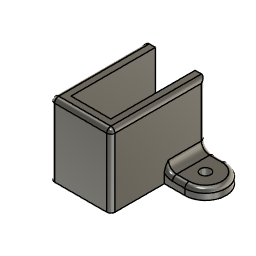
Motor Mount v1 (Autodesk Fusion 360 design; units mm, degrees)
Autodesk Fusion 360 part; units mm, degrees
sketch "Sketch1" plane through (0, 0, 0) normal (0, 0, 1) x (1, 0, 0)
  line L0 (0, 0) -> (12.2682, 0)
  line L1 (12.2682, 0) -> (12.2682, 22.86)
  line L2 (12.2682, 22.86) -> (0, 22.86)
  line L3 (0, 22.86) -> (0, 0)
  line L4 (-3.175, -3.175) -> (15.4432, -3.175)
  line L5 (15.4432, -3.175) -> (15.4432, 26.035)
  line L6 (15.4432, 26.035) -> (-3.175, 26.035)
  line L7 (-3.175, 26.035) -> (-3.175, -3.175)
  line L8 (0, 22.86) -> (0, 26.035)
  line L9 (12.2682, 22.86) -> (12.2682, 26.035)
  dimension "d1" = 12.2682
  dimension "d2" = 22.86
  dimension "d3" = 3.175
  constraint horizontal L0
  constraint vertical L1
  constraint horizontal L2
  constraint vertical L3
  constraint coincident L0.start L3.end
  constraint coincident L6 L8.end
  constraint perpendicular L6 L8
  constraint coincident L6 L9.end
  constraint perpendicular L6 L9
  measures "d1" distance of L0.start L0.end
  measures "d2" distance of L0.start L2.end
extrude "Extrude1" add sketch "Sketch1" along normal blind 3.175
sketch "Sketch2" plane through (0, 0, 3.175) normal (0, 0, 1) x (-1, 0, 0)
  line L0 (3.175, -26.035) -> (3.175, 3.175)
  line L1 (3.175, 3.175) -> (-15.4432, 3.175)
  line L2 (-15.4432, 3.175) -> (-15.4432, -26.035)
  line L3 (-15.4432, -26.035) -> (3.175, -26.035)
  line L4 (-12.2682, 0) -> (-12.2682, -22.86)
  line L5 (-12.2682, -22.86) -> (0, -22.86)
  line L6 (0, -22.86) -> (0, 0)
  line L7 (0, 0) -> (-12.2682, 0)
  dimension "d6" = -3.175
extrude "Extrude2" add sketch "Sketch2" along normal blind 3.175
sketch "Sketch3" plane through (0, 0, 6.35) normal (0, 0, 1) x (-1, 0, 0)
  line L0 (-12.2682, 0) -> (0, 0)
  line L1 (0, 0) -> (0, -22.86)
  line L2 (0, -22.86) -> (-12.2682, -22.86)
  line L3 (-12.2682, -22.86) -> (-12.2682, 0)
  line L4 (-15.4432, -26.035) -> (3.175, -26.035)
  line L5 (3.175, -26.035) -> (3.175, 3.175)
  line L6 (3.175, 3.175) -> (-15.4432, 3.175)
  line L7 (-15.4432, 3.175) -> (-15.4432, -26.035)
  line L8 (0, -22.86) -> (0, -26.035)
  line L9 (-12.2682, -22.86) -> (-12.2682, -26.035)
  constraint coincident L1.end L2.start
  constraint coincident L4 L8.end
  constraint perpendicular L4 L8
  constraint coincident L2.end L3.start
  constraint coincident L4 L9.end
  constraint perpendicular L4 L9
extrude "Extrude3" add sketch "Sketch3" along normal blind 16.002 contours L0 L1 L3 L4 L5 L6 L7 L8 L9
sketch "Sketch4" plane through (0, 0, 0) normal (0, 0, -1) x (1, 0, 0)
  line L0 (-3.175, 3.175) -> (-3.175, -26.035)
  line L1 (-3.175, -26.035) -> (15.4432, -26.035)
  line L2 (15.4432, -26.035) -> (15.4432, 3.175)
  line L3 (15.4432, 3.175) -> (-3.175, 3.175)
  line L4 (15.4432, -26.035) -> (21.7932, -26.035)
  line L5 (21.7932, -26.035) -> (21.7932, -19.685)
  line L6 (21.7932, -19.685) -> (15.4432, -19.685)
  line L7 (15.4432, -19.685) -> (15.4432, -26.035)
  line L8 (-3.175, -26.035) -> (-9.525, -26.035)
  line L9 (-9.525, -26.035) -> (-9.525, -19.685)
  line L10 (-9.525, -19.685) -> (-3.175, -19.685)
  line L11 (-3.175, -19.685) -> (-3.175, -26.035)
  circle A0 centre (21.7932, -19.685) radius 6.35
  circle A1 centre (-9.525, -19.685) radius 6.35
  line L12 (-9.525, -19.685) -> (21.7932, -19.685)
  line L13 (21.7932, -19.685) -> (21.7932, -13.335)
  line L14 (21.7932, -13.335) -> (-9.525, -13.335)
  line L15 (-9.525, -13.335) -> (-9.525, -19.685)
  dimension "d11" = 6.35
  dimension "d12" = 6.35
  dimension "d13" = 6.35
  dimension "d14" = 6.35
  constraint horizontal L4
  constraint vertical L5
  constraint horizontal L6
  constraint vertical L7
  constraint coincident L1.end L2.start
  constraint horizontal L8
  constraint vertical L9
  constraint horizontal L10
  constraint vertical L11
  constraint coincident L0.end L1.start
  constraint coincident L5.end L6.start
  constraint coincident L4.end A0
  constraint coincident L9.end L10.start
  constraint coincident L8.end A1
  constraint horizontal L12
  constraint vertical L13
  constraint horizontal L14
  constraint vertical L15
  constraint coincident A0 L13.end
  measures "d11" distance of L1.end L4.end
  measures "d12" distance of L1.end L6.end
  measures "d13" distance of L0.end L8.end
  measures "d14" distance of L0.end L10.end
extrude "Extrude4" add sketch "Sketch4" against normal blind 3.175 contours L0 A1 L14 | L9 L10 A1 L12 | L10 A1 L12 L15 | L0 L8 L11 A1 | L9 A1 L15 | L2 L4 L7 A0 | L6 A0 L12 L13 | L2 A0 L14 | L5 L6 A0 L12 | L5 A0 L13
sketch "Sketch5" plane through (0, 0, 3.175) normal (0, 0, 1) x (-1, 0, 0)
  line L0 (-15.4432, -26.035) -> (-15.4432, -13.335)
  line L1 (-15.4432, -13.335) -> (-21.7932, -13.335)
  arc A0 (-21.7932, -13.335) -> (-21.7932, -26.035) centre (-21.7932, -19.685) ccw
  line L2 (-21.7932, -26.035) -> (-15.4432, -26.035)
  circle A1 centre (-21.7932, -19.685) radius 1.5875
  dimension "d17" = 3.175
  constraint concentric A0 A1
  measures "d17" diameter of A1
extrude "Extrude5" cut sketch "Sketch5" against normal blind 127 contours A1
sketch "Sketch6" plane through (0, 0, 3.175) normal (0, 0, 1) x (-1, 0, 0)
  arc A0 (9.525, -26.035) -> (9.525, -13.335) centre (9.525, -19.685) ccw
  line L0 (9.525, -13.335) -> (3.175, -13.335)
  line L1 (3.175, -13.335) -> (3.175, -26.035)
  line L2 (3.175, -26.035) -> (9.525, -26.035)
  circle A1 centre (9.525, -19.685) radius 1.5875
  dimension "d20" = 3.175
  constraint concentric A0 A1
  measures "d20" diameter of A1
extrude "Extrude6" cut sketch "Sketch6" against normal blind 25.4 contours A1
fillet "Fillet1" radius 2.54 1 edges at (15.4432, 19.685, 3.175)
fillet "Fillet2" radius 2.54 1 edges at (-3.175, 19.685, 3.175)
fillet "Fillet3" radius 1.27 17 edges at (-3.175, 11.43, 22.352) (-3.9189, 13.335, 3.9189) (-7.62, 13.335, 3.175) (-15.875, 19.685, 3.175) (-7.62, 26.035, 3.175) (-3.9189, 26.035, 3.9189) (-3.175, 26.035, 14.0335) (-3.175, -3.175, 11.176) (15.4432, -3.175, 11.176) (6.1341, -3.175, 22.352) (15.4432, 11.43, 22.352) (16.1871, 13.335, 3.9189) (19.8882, 13.335, 3.175) (28.1432, 19.685, 3.175) (19.8882, 26.035, 3.175) (16.1871, 26.035, 3.9189) (15.4432, 26.035, 14.0335)
